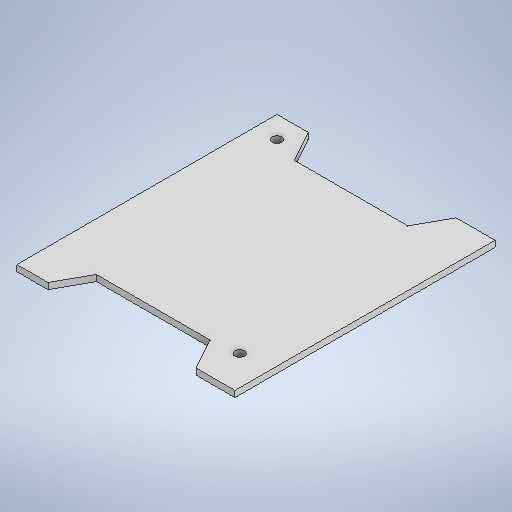
# Autodesk Inventor part: plytka
Saved by Autodesk Inventor 2025 (Build 290162000, 162)
## iProperties
Created: 2025-03-18
Part Number: plytka
Material: Generic
Document SubType Name: Modeling
Designer: HP
Density: 1 g/cm^3
Appearance: Default
Author: HP
Autodesk Inventor part; units mm, degrees
ref_plane "YZ Plane" through (0, 0, 0) normal (1, 0, 0) x (0, 1, 0)
ref_plane "XZ Plane" through (0, 0, 0) normal (0, 1, 0) x (-1, 0, 0)
ref_plane "XY Plane" through (0, 0, 0) normal (0, 0, 1) x (1, 0, 0)
sketch "Sketch1" plane through (0, 0, 0) normal (0, 1, 0) x (-1, 0, 0)
  line L0 (0, -41.75) -> (0, -83.5)
  line L1 (0, -83.5) -> (12.5, -83.5)
  line L2 (18, -73.5) -> (54.5, -73.5)
  line L3 (70, -83.5) -> (70, -41.75)
  line L4 (70, -83.5) -> (60, -83.5)
  line L5 (60, -83.5) -> (54.5, -73.5)
  line L6 (18, -73.5) -> (12.5, -83.5)
  line L7 (0, -41.75) -> (0, 0)
  line L8 (0, 0) -> (12.5, 0)
  line L9 (18, -10) -> (54.5, -10)
  line L10 (70, 0) -> (70, -41.75)
  line L11 (70, 0) -> (60, 0)
  line L12 (60, 0) -> (54.5, -10)
  line L13 (18, -10) -> (12.5, 0)
  constraints: 28 end point, 2 point on line, 1 perpendicular, 1 vertical
extrude "Extrusion1" add sketch "Sketch1" along normal blind 2
sketch "Sketch3" plane through (0, 2, 0) normal (0, 1, 0) x (1, 0, 0)
  circle A0 centre (-9.5, 11) radius 1.5
  line L0 (-60, 83.5) -> (-70, 83.5) projected
  line L1 (-70, 83.5) -> (-63, 83.5)
  line L2 (-70, 83.5) -> (-63, 83.5)
  line L3 (-70, 83.5) -> (-63, 83.5)
  line L4 (-63, 83.5) -> (-63, 76.5)
  circle A1 centre (-63, 76.5) radius 1.5
  point P0 (0, 0)
  dimension "d10" = 3
  dimension "d11" = 7
  dimension "d12" = 7
  dimension "d13" = 3
  constraints: 8 end point, 2 centre point, 2 collinear, 1 coincident, 1 point on line, 1 vertical
  measures "d10" diameter of A0
  measures "d11" distance of L0.end L1.end
  measures "d12" distance of L1.end L4.end
  measures "d13" diameter of A1
extrude "Extrusion2" cut sketch "Sketch3" against normal blind 10
body "Solid1"
